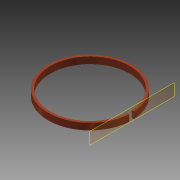
# Autodesk Inventor part: ringLoop
Saved by Autodesk Inventor 2015 (Build 190159000, 159)
## iProperties
Created: 2014-05-20
Part Number: ringLoop
Material: Copper
Document SubType Name: Modeling
Designer: jad211
Density: 8.94 g/cm^3
Appearance: Copper - Satin
Author: jad211
Autodesk Inventor part; units mm, degrees
ref_plane "XZ Plane" through (0, 0, 0) normal (0, 1, 0) x (-1, 0, 0)
ref_plane "XY Plane" through (0, 0, 0) normal (0, 0, 1) x (1, 0, 0)
sketch "Sketch1" plane through (0, 0, 0) normal (0, 1, 0) x (-1, 0, 0)
  circle A0 centre (0, 0) radius 19
  circle A1 centre (0, 0) radius 18
  dimension "d0" = 38
  dimension "d1" = 36
  constraints: 2 centre point, 2 coincident
  measures "d0" diameter of A0
  measures "d1" diameter of A1
extrude "Extrusion1" add sketch "Sketch1" along normal blind 3
ref_plane "Work Plane1" through (19, 0, 0) normal (1, 0, 0) x (0, 1, 0)
sketch "Sketch2" plane through (19, 0, 0) normal (1, 0, 0) x (0, 1, 0)
  line L0 (0, 1) -> (5, 1)
  line L1 (5, 1) -> (5, -1)
  line L2 (5, -1) -> (0, -1)
  line L3 (0, -1) -> (0, 1)
  point P0 (0, 0)
  dimension "d4" = 1
  dimension "d5" = 1
  dimension "d6" = 0
  dimension "d7" = 5
  constraints: 8 end point
  measures "d4" distance from line of point (0, 0) L0
  measures "d5" distance from line of point (0, 0) L2
  measures "d6" distance from line of point (0, 0) L3
  measures "d7" distance between parallel lines of L3 L1
extrude "Extrusion2" cut sketch "Sketch2" against normal blind 5
equation "\"d5\" = d4"
body "Solid1"
